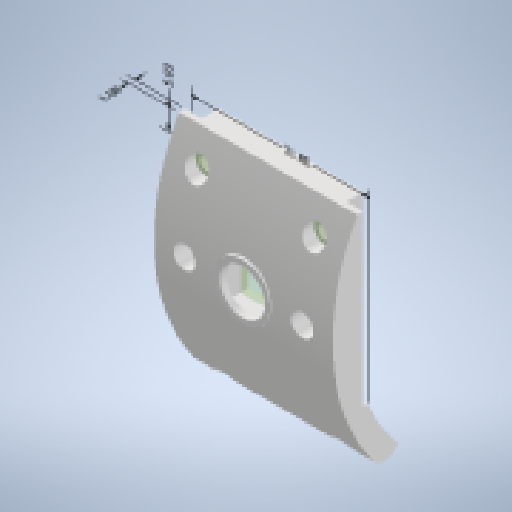
# Autodesk Inventor part: cover_front
Saved by Autodesk Inventor 2024.1 (Build 281209000, 209)
## iProperties
Created: 2025-01-10
Part Number: cover_front
Material: 一般
Document SubType Name: Modeling
Designer: hibik
Density: 1 g/cm^3
Appearance: 既定
Author: hibik
Autodesk Inventor part; units mm, degrees
ref_plane "YZ Plane" through (0, 0, 0) normal (1, 0, 0) x (0, 1, 0)
ref_plane "XZ Plane" through (0, 0, 0) normal (0, 1, 0) x (-1, 0, 0)
ref_plane "XY Plane" through (0, 0, 0) normal (0, 0, 1) x (1, 0, 0)
sketch "スケッチ1" plane through (0, 0, 0) normal (0, 0, 1) x (1, 0, 0)
  line L0 (12.9, 14.6391) -> (-12.9, 14.6391)
  line L1 (-12.9, 14.6391) -> (-12.9, -9.7609)
  line L2 (-12.9, -9.7609) -> (12.9, -9.7609)
  line L3 (12.9, -9.7609) -> (12.9, 14.6391)
  line L4 (12.9, 14.6391) -> (-12.9, -9.7609) construction
  line L5 (-12.9, 14.6391) -> (12.9, -9.7609) construction
  line L6 (12.7, -9.5717) -> (-12.7, -9.5717) construction
  line L7 (-12.7, -9.5717) -> (-12.7, 14.45) construction
  line L8 (-12.7, 14.45) -> (12.7, 14.45) construction
  line L9 (12.7, 14.45) -> (12.7, -9.5717) construction
  line L10 (12.7, -9.5717) -> (-12.7, 14.45) construction
  line L11 (-12.7, -9.5717) -> (12.7, 14.45) construction
  line L12 (15.9, -12.5981) -> (-15.9, -12.5981)
  line L13 (-15.9, -12.5981) -> (-15.9, 17.4764)
  line L14 (-15.9, 17.4764) -> (15.9, 17.4764)
  line L15 (15.9, 17.4764) -> (15.9, -12.5981)
  line L16 (15.9, -12.5981) -> (-15.9, 17.4764) construction
  line L17 (-15.9, -12.5981) -> (15.9, 17.4764) construction
  line L18 (10.5, -0.05) -> (-10.5, -0.05) construction
  line L19 (-10.5, -0.05) -> (-10.5, 12.45) construction
  line L20 (-10.5, 12.45) -> (10.5, 12.45) construction
  line L21 (10.5, 12.45) -> (10.5, -0.05) construction
  line L22 (10.5, -0.05) -> (-10.5, 12.45) construction
  line L23 (-10.5, -0.05) -> (10.5, 12.45) construction
  circle A0 centre (10.5, 12.45) radius 1.2
  circle A1 centre (-10.5, 12.45) radius 1.2
  circle A2 centre (10.5, -0.05) radius 1.2
  circle A3 centre (-10.5, -0.05) radius 1.2
  line L24 (4.5, 4.5) -> (-4.5, 4.5)
  line L25 (-4.5, 4.5) -> (-4.5, -4.5)
  line L26 (-4.5, -4.5) -> (4.5, -4.5)
  line L27 (4.5, -4.5) -> (4.5, 4.5)
  line L28 (4.5, 4.5) -> (-4.5, -4.5) construction
  line L29 (-4.5, 4.5) -> (4.5, -4.5) construction
  line L30 (-6.5, 4.5) -> (6.5, 4.5)
  line L31 (6.5, 4.5) -> (6.5, 12)
  line L32 (6.5, 12) -> (-6.5, 12)
  line L33 (-6.5, 12) -> (-6.5, 4.5)
  line L34 (12.9, -9.7609) -> (12.9, -12.9)
  line L35 (-12.9, -9.7609) -> (-12.9, -12.5981)
  line L36 (12.9, 14.6391) -> (12.9, 17.4764)
  line L37 (-12.9, 14.6391) -> (-12.9, 17.4764)
  point P0 (0, 0)
  point P1 (0, 2.4391)
  point P2 (0, 6.2)
  point P3 (0, 12)
  point P4 (12.9, -12.5981)
  dimension "d0" = 25.8
  dimension "d1" = 24.4
  dimension "d2" = 25.4
  dimension "d3" = 14.45
  dimension "d4" = 3
  dimension "d5" = 21
  dimension "d6" = 12.5
  dimension "d7" = 2
  dimension "d8" = 2.4
  dimension "d12" = 9
  dimension "d13" = 9
  dimension "d14" = 13
  dimension "d15" = 7.5
  constraints: 76 end point, 12 parallel, 11 midpoint, 8 perpendicular, 8 point on line, 6 horizontal, 4 centre point, 4 coincident, 3 equal radius, 3 vertical alignment
  measures "d0" distance of L0.start L0.end
  measures "d1" distance of L0.end L1.end
  measures "d2" distance of L7.end L8.end
  measures "d3" distance from line of L8 point (0, 0)
  measures "d4" distance between parallel lines of L13 L1
  measures "d5" distance of L19.end L20.end
  measures "d6" distance of L18.end L19.end
  measures "d7" distance between parallel lines of L8 L20
  measures "d8" diameter of A0
  measures "d12" distance of L26.end L25.end
  measures "d13" distance of L25.end L24.end
  measures "d14" distance of L32.end L31.end
  measures "d15" distance of L31.end L30.end
extrude "押し出し1" add sketch "スケッチ1" along normal blind 4.5 contours L3 L2 L1 L0 | L36 L14 L15 L12 L34 L3 | L0 L37 L14 L36 | L1 L35 L12 L13 L14 L37 | L34 L12 L35 L2 | L24 L30 L33 L32 L31
extrude "押し出し4" cut sketch "スケッチ1" along normal blind 2 contours L24 L30 L33 L32 L31
sketch "スケッチ4" plane through (0, 0, 4.5) normal (0, 0, 1) x (1, 0, 0)
  line L0 (15.9, 17.4764) -> (-15.9, 17.4764) projected
  line L1 (-15.9, 17.4764) -> (-15.9, -12.5981) projected
  line L2 (-15.9, -12.5981) -> (15.9, -12.5981) projected
  line L3 (15.9, -12.5981) -> (15.9, 17.4764) projected
  line L4 (4.5, -4.5) -> (-4.5, -4.5) projected
  line L5 (-4.5, -4.5) -> (-4.5, 4.5) projected
  line L6 (-4.5, 4.5) -> (4.5, 4.5) projected
  line L7 (4.5, 4.5) -> (4.5, -4.5) projected
  circle A0 centre (-10.5, -0.05) radius 1.2 projected
  circle A1 centre (10.5, -0.05) radius 1.2 projected
  circle A2 centre (-10.5, 12.45) radius 1.2 projected
  circle A3 centre (10.5, 12.45) radius 1.2 projected
  circle A4 centre (0, 0) radius 4
  dimension "d24" = 8
  constraints: 1 centre point, 1 coincident
  measures "d24" diameter of A4
extrude "押し出し5" add sketch "スケッチ4" along normal blind 1 contours L3 L2 L1 L0 | L4 L5 L6 L7
sketch "スケッチ5" plane through (-15.9, -12.5981, 0) normal (-1, 0, 0) x (0, 0, 1)
  arc A0 (-14.875, -15.7643) -> (-2.8877, 28.9731) centre (-31.25, 12.5981) ccw projected
  circle A1 centre (-31.25, 12.5981) radius 36.75
  line L0 (0, 30.0744) -> (0, 0) projected
  line L1 (0, 0) -> (5.5, 0) projected
  line L2 (5.5, 30.0744) -> (5.5, 0) projected
  line L3 (0, 30.0744) -> (5.5, 30.0744) projected
  line L4 (5.5, 30.0744) -> (5.5, 0) projected
  point P0 (0, 12.5981)
  point P1 (1.0786, 30.0744)
  point P2 (5.5, 12.5981)
  point P3 (3.2732, 0)
  constraints: 1 centre point, 1 coincident, 1 tangent
extrude "押し出し6" cut sketch "スケッチ5" against normal through all contours A1 L2 L1 | L3 L2 A1
extrude "押し出し7" add sketch "スケッチ1" against normal blind 3 contours L0 L37 L14 L36
ref_plane "作業平面1" through (0, 0, 1.5) normal (0, 0, -1) x (-1, 0, 0)
sketch "スケッチ7" plane through (0, 0, 1.5) normal (0, 0, -1) x (-1, 0, 0)
  circle A0 centre (-10.5, -0.05) radius 1.1 projected
  circle A1 centre (10.5, -0.05) radius 1.2 projected
  circle A2 centre (10.5, 12.45) radius 1.2 projected
  circle A3 centre (-10.5, 12.45) radius 1.1 projected
  circle A4 centre (-10.5, 12.45) radius 2
  circle A5 centre (-10.5, -0.05) radius 2
  circle A6 centre (10.5, -0.05) radius 2
  circle A7 centre (10.5, 12.45) radius 2
  point P0 (0, 0)
  dimension "d47" = 4
  constraints: 4 centre point, 4 coincident, 3 equal radius, 3 horizontal alignment, 2 other
  measures "d47" diameter of A4
extrude "押し出し8" cut sketch "スケッチ7" against normal through all contours A0 | A1 | A2 | A3 | A4 | A5 | A6 | A7
sketch "スケッチ8" plane through (-15.9, -12.5981, -3) normal (-1, 0, 0) x (0, 0, 1)
  line L0 (-3.4563, -8.799) -> (-8.3519, -4.5741) projected
  arc A0 (-11.875, -15.7643) -> (0.1123, 28.9731) centre (-28.25, 12.5981) ccw projected
  arc A1 (6.2732, 0) -> (4.0786, 30.0744) centre (-28.25, 12.5981) ccw projected
  circle A2 centre (-28.25, 12.5981) radius 36.75
  line L1 (-3.4563, -8.799) -> (-0.4281, -11.4124)
  circle A3 centre (-28.25, 12.5981) radius 32.95
  line L2 (3, 0) -> (6.2732, 0) projected
  line L3 (3, 0) -> (1.98, 0)
  point P0 (3, 12.5981)
  point P1 (0, 0)
  point P2 (6.2732, 0)
  point P3 (2.1965, 0)
  point P4 (-3.3049, -8.9297)
  point P5 (4.0786, 30.0744)
  point P6 (2.1965, 0)
  dimension "d50" = 0.2
  constraints: 4 end point, 2 coincident, 1 centre point, 1 horizontal, 1 point on circle, 1 point on line, 4 other
  measures "d50" radial gap between concentric circles of A3 A0
extrude "押し出し9" add sketch "スケッチ8" against normal up to surface (31.8 mm away) contours A3 L3 L2 A2 L1
sketch "スケッチ9" plane through (0, 0, 4.5) normal (0, 0, -1) x (-1, 0, 0)
  circle A0 centre (0, 0) radius 4 projected
  circle A1 centre (0, 0) radius 5
  dimension "d53" = 10
  constraints: 1 centre point, 1 coincident
  measures "d53" diameter of A1
extrude "押し出し10" add sketch "スケッチ9" against normal blind 1.2
ref_plane "作業平面2" through (-10.5, -16.5887, -8.9111) normal (0, -0.6533458, 0.7570597) x (1, 0, 0)
sketch "スケッチ10" plane through (-10.5, -16.5887, -8.9111) normal (0, -0.6533458, 0.7570597) x (1, 0, 0)
  line L0 (-5.4, 2.0364) -> (-5.4, 1.7877) projected
  circle A0 centre (0, 0) radius 0.9 projected
  circle A1 centre (0, 0) radius 1.2
  point P0 (10.5, 18.3806)
  dimension "d56" = 2.4
  constraints: 1 centre point, 1 coincident
  measures "d56" diameter of A1
extrude "押し出し11" cut sketch "スケッチ10" along normal through all contours A0 | A1
ref_plane "作業平面3" through (-10.5, -20.8354, -3.9902) normal (0, -0.6533458, 0.7570597) x (1, 0, 0)
sketch "スケッチ11" plane through (-10.5, -20.8354, -3.9902) normal (0, -0.6533458, 0.7570597) x (1, 0, 0)
  circle A0 centre (0, 0) radius 2
  circle A1 centre (0, 0) radius 0.9 projected
  point P0 (10.5, 18.3806)
  dimension "d60" = 4
  constraints: 1 centre point, 1 concentric
  measures "d60" diameter of A0
extrude "押し出し12" cut sketch "スケッチ11" along normal through all
mirror "ミラー1" about plane through (0, 0, 0) normal (1, 0, 0) of "押し出し11", "押し出し12"
fillet "フィレット2" radius 2.5 1 edges at (0, -24.0105, -3.4281)
